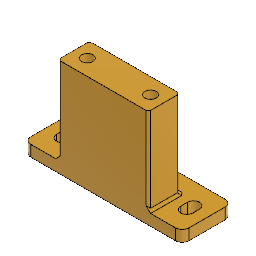
power_mount v8 (Autodesk Fusion 360 design; units mm, degrees)
Autodesk Fusion 360 part; units mm, degrees
sketch "Sketch1" plane through (0, 0, 0) normal (0, 0, 1) x (1, 0, 0)
  line L0 (20, -11) -> (-20, -11)
  line L1 (-20, -11) -> (-20, 11)
  line L2 (-20, 11) -> (20, 11)
  line L3 (20, 11) -> (20, -11)
  line L4 (20, -11) -> (-20, 11) construction
  line L5 (-20, -11) -> (20, 11) construction
  line L6 (20, 11) -> (35, 11)
  line L7 (35, 11) -> (35, -11)
  line L8 (35, -11) -> (20, -11)
  line L9 (20, -11) -> (20, 11)
  line L10 (-20, 11) -> (-35, 11)
  line L11 (-35, 11) -> (-35, -11)
  line L12 (-35, -11) -> (-20, -11)
  line L13 (-20, -11) -> (-20, 11)
  line L14 (-35, 0) -> (35, 0)
  circle A0 centre (27.5, 0) radius 2.65
  circle A1 centre (27.5, 0) radius 5.5 construction
  line L15 (27.5, 11) -> (27.5, -11) construction
  line L16 (-27.5, 11) -> (-27.5, -11) construction
  circle A2 centre (-27.5, 0) radius 2.65
  line L17 (-20, 3) -> (20, 3)
  line L18 (-20, -4) -> (20, -4) construction
  circle A3 centre (14, -4) radius 2.55
  circle A4 centre (-14, -4) radius 2.55
  line L19 (-35, 1.5) -> (35, 1.5) construction
  line L20 (-35, -1.5) -> (35, -1.5) construction
  circle A5 centre (-27.5, 1.5) radius 2.65
  circle A6 centre (-27.5, -1.5) radius 2.65
  circle A7 centre (27.5, -1.5) radius 2.65
  circle A8 centre (27.5, 1.5) radius 2.65
  line L21 (24.85, 1.5) -> (24.85, -1.5)
  line L22 (30.15, 1.5) -> (30.15, -1.5)
  line L23 (-30.15, 1.5) -> (-30.15, -1.5)
  line L24 (-24.85, 1.5) -> (-24.85, -1.5)
  dimension "d1" = 22
  dimension "d2" = 40
  dimension "d3" = 15
  dimension "d4" = 15
  dimension "d5" = 5.3
  dimension "d6" = 11
  dimension "d7" = 5.3
  dimension "d21" = 14
  dimension "d22" = 7
  dimension "d23" = 5.1
  dimension "d24" = 5.1
  dimension "d25" = 6
  dimension "d26" = 6
  dimension "d32" = 1.5
  dimension "d33" = 1.5
  dimension "d34" = 5.3
  dimension "d35" = 5.3
  dimension "d36" = 5.3
  dimension "d37" = 5.3
  dimension "d40" = 28
  dimension "d41" = 55
  dimension "d42" = 13.5
  constraint perpendicular L0 L1
  constraint parallel L0 L2
  constraint parallel L1 L3
  constraint horizontal L0
  constraint coincident L4 origin
  constraint coincident L5 origin
  constraint horizontal L6
  constraint vertical L7
  constraint horizontal L8
  constraint vertical L9
  constraint horizontal L10
  constraint vertical L11
  constraint horizontal L12
  constraint vertical L13
  constraint collinear L0 L12
  constraint collinear L0 L8
  constraint midpoint L11 L14.start
  constraint midpoint L7 L14.end
  constraint coincident L14 A0.centre
  constraint concentric A0 A1
  constraint midpoint L6 L15.start
  constraint midpoint L8 L15.end
  constraint coincident A0.centre L15
  constraint midpoint L10 L16.start
  constraint midpoint L12 L16.end
  constraint midpoint L16 A2.centre
  constraint coincident L1 L17.start
  constraint coincident L3 L17.end
  constraint perpendicular L13 L17
  constraint coincident L13 L18.start
  constraint coincident L3 L18.end
  constraint perpendicular L13 L18
  constraint coincident L18 A3.centre
  constraint coincident L18 A4.centre
  constraint coincident L11 L19.start
  constraint coincident L7 L19.end
  constraint perpendicular L7 L19
  constraint coincident L11 L20.start
  constraint coincident L7 L20.end
  constraint perpendicular L7 L20
  constraint coincident L19 A5.centre
  constraint coincident L16 A5.centre
  constraint coincident L16 A6.centre
  constraint coincident L20 A6.centre
  constraint coincident L15 A7.centre
  constraint coincident L20 A7.centre
  constraint coincident L19 A8.centre
  constraint coincident L15 A8.centre
  constraint coincident L19 L21.start
  constraint coincident A8 L21.start
  constraint coincident L20 L21.end
  constraint coincident A7 L21.end
  constraint coincident L19 L22.start
  constraint coincident A8 L22.start
  constraint coincident L20 L22.end
  constraint coincident A7 L22.end
  constraint coincident L19 L23.start
  constraint coincident A5 L23.start
  constraint coincident L20 L23.end
  constraint coincident A6 L23.end
  constraint coincident L19 L24.start
  constraint coincident A5 L24.start
  constraint coincident L20 L24.end
  constraint coincident A6 L24.end
  measures "d1" distance of L0 L2
  measures "d2" distance of L1.end L2.end
  measures "d3" distance of L2.end L6.end
  measures "d4" distance of L1.end L10.end
  measures "d5" diameter of A0
  measures "d6" diameter of A1
  measures "d7" diameter of A2
  measures "d21" distance of L0 L17
  measures "d22" distance of L17 L18
  measures "d23" diameter of A3
  measures "d24" diameter of A4
  measures "d25" distance of L9 A3.centre
  measures "d26" distance of L13 A4.centre
  measures "d32" distance of L14 L19
  measures "d33" distance of L14 L20
  measures "d34" diameter of A5
  measures "d35" diameter of A6
  measures "d36" diameter of A7
  measures "d37" diameter of A8
  measures "d40" distance of A3.centre A4.centre
  measures "d41" distance of A0.centre A2.centre
  measures "d42" horizontal distance of A2.centre A4.centre
extrude "Extrude2" add sketch "Sketch1" along normal blind 43.5 contours L0 L1 L3 L9 L13 L14 | L1 L3 L9 L13 L14 L17 | A3 | A4
extrude "Extrude1" add sketch "Sketch1" along normal blind 5 contours L3 L7 L8 L9 L14 A7 L21 L22 | L1 L11 L12 L13 L14 A6 L23 L24 | L3 L6 L7 L9 L14 A8 L21 L22 | L1 L10 L11 L13 L14 A5 L23 L24 | L1 L2 L3 L9 L13 L17
extrude "Extrude4" cut sketch "Sketch1" against normal blind 10 from surface at 43.5 contours A3 | A4
fillet "Fillet3" radius 3 4 edges at (-35, -11, 2.5) (-35, 11, 2.5) (35, 11, 2.5) (35, -11, 2.5)
chamfer "Chamfer2" distance 1 angle 45 3 edges at (20, -4, 5) (0, 3, 5) (-20, -4, 5)
chamfer "Chamfer3" distance 1 angle 45 6 edges at (20, -11, 24.75) (20, 3, 24.75) (-20, 3, 24.75) (-20, -11, 24.75) (-20.5, 3.5, 5.5) (20.5, 3.5, 5.5)
chamfer "Chamfer1" [suppressed]
equation "d4 = d3"
equation "d7 = d5"
equation "d22 = ( d21 ) / 2"
equation "d24 = d23"
equation "d26 = d25"
equation "d33 = d32"
equation "d34 = d5"
equation "d35 = d5"
equation "d36 = d5"
equation "d37 = d5"
